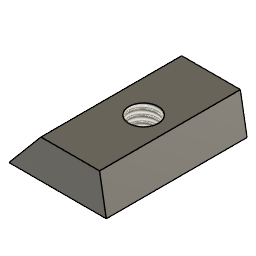
Wedge (Autodesk Fusion 360 design; units mm, degrees)
Autodesk Fusion 360 part; units mm, degrees
ref_plane "WorkPlane1" through (0, 0, 0.4062) normal (0, 0, 1) x (1, 0, 0)
sketch "Sketch1" plane through (0, 0, 0.4062) normal (0, 0, 1) x (1, 0, 0)
  line L0 (0, 0) -> (0.625, 0)
  line L1 (0.625, 0) -> (0.625, 1.5)
  line L2 (0.625, 1.5) -> (0, 1.5)
  line L3 (0, 1.5) -> (0, 0)
  dimension "d2" = 0.625
  dimension "d3" = 1.5
  constraint horizontal L0
  constraint vertical L1
  constraint horizontal L2
  constraint vertical L3
  constraint coincident L0.start L3.end
  measures "d2" distance of L0.start L0.end
  measures "d3" distance of L0.start L2.end
sketch "Sketch2" plane through (0, 0, 0) normal (0, 1, 0) x (1, 0, 0)
  line L0 (0, 0) -> (0, -0.4062)
  line L1 (0, -0.4062) -> (-0.3409, 0)
  line L2 (0, -0.4062) -> (-0.632, -0.4062) construction
  line L3 (-0.3409, 0) -> (-0.21, 0)
  line L4 (0, -0.4062) -> (0.625, -0.4062)
  line L5 (0.625, -0.4062) -> (0.6966, 0)
  line L6 (0.6966, 0) -> (0, 0)
  line L7 (0, 0) -> (-0.3409, 0)
  dimension "d4" = 0.4063
  dimension "d5" = 50
  dimension "d6" = 0.625
  dimension "d7" = 80
  constraint coincident L0.start L6.end
  constraint vertical L0
  constraint horizontal L2
  constraint perpendicular L0 L3
  constraint perpendicular L0 L4
  measures "d4" distance of L0.start L0.end
  measures "d5" angle of L1 L2
  measures "d6" distance of L0.end L4.end
  measures "d7" angle of L4 L5
extrude "Extrude1" add sketch "Sketch2" along normal blind 1.5
hole "Hole1" at (0.3438, 0.75, 0.4062) direction (0, 0, -1) diameter 0.375 depth 0.41 tip angle 180
scale "Scale1" factor 25.4 about (0, 0, 0.4062) bodies 1
thread "Thread2" "ANSI Unified Screw Threads 0.375 3/8-16 UNC 3/8-16 UNC 3B" major diameter 9.525 minor diameter 7.94 pitch 1.5875 angle 60 resizes the face on face at (9.2054, 14.3112, -6.4728)
